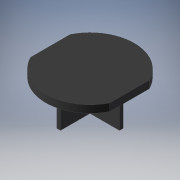
# Autodesk Inventor part: Syringe cap_Flat_Sides
Saved by Autodesk Inventor 2019 (Build 230136000, 136)
## iProperties
Created: 2019-01-24
Part Number: Syringe cap_Flat_Sides
Material: Generic
Document SubType Name: Modeling
Designer: dewanlab
Density: 1 g/cm^3
Appearance: Default
Author: dewanlab
Autodesk Inventor part; units mm, degrees
ref_plane "YZ Plane" through (0, 0, 0) normal (1, 0, 0) x (0, 1, 0)
ref_plane "XZ Plane" through (0, 0, 0) normal (0, 1, 0) x (-1, 0, 0)
ref_plane "XY Plane" through (0, 0, 0) normal (0, 0, 1) x (1, 0, 0)
sketch "Sketch1" plane through (0, 0, 0) normal (0, 1, 0) x (-1, 0, 0)
  line L0 (-17.05, 0) -> (-17.05, 8.4971)
  line L1 (-17.05, 0) -> (-17.05, -8.4971)
  line L2 (17.05, 0) -> (17.05, 8.4971)
  line L3 (17.05, 0) -> (17.05, -8.4971)
  arc A0 (-17.05, -8.4971) -> (17.05, -8.4971) centre (0, 0) ccw
  arc A1 (17.05, 8.4971) -> (-17.05, 8.4971) centre (0, 0) ccw
  constraints: 8 end point, 4 point on circle, 2 centre point, 2 point on line, 1 coincident
extrude "Extrusion1" add sketch "Sketch1" along normal blind 3.175
sketch "Sketch4" plane through (0, 0, 0) normal (0, -1, 0) x (-1, 0, 0)
  line L0 (-13.4937, -0.7938) -> (13.4938, -0.7938)
  line L1 (13.4938, -0.7938) -> (13.4938, 0.7938)
  line L2 (13.4938, 0.7938) -> (-13.4938, 0.7937)
  line L3 (-13.4938, 0.7937) -> (-13.4937, -0.7938)
  circle A0 centre (0, 0) radius 19.05 projected
  dimension "d16" = 26.9875
  dimension "d17" = 1.5875
  dimension "d18" = 18.2563
  dimension "d19" = 5.5563
  constraints: 8 end point, 2 parallel, 1 horizontal, 1 perpendicular
  measures "d16" distance of L1.end L2.end
  measures "d17" distance of L2.end L0.start
  measures "d18" distance edge to line of A0 L2
  measures "d19" distance edge to line of A0 L3
extrude "Extrusion3" add sketch "Sketch4" along normal blind 12.7 contours L3 L2 L1 L0
sketch "Sketch5" plane through (0, 0, 0) normal (0, -1, 0) x (-1, 0, 0)
  line L0 (13.4937, 0.7938) -> (-13.4938, 0.7937) projected
  line L1 (-0.7938, 0.7937) -> (0.6758, 0.7937)
  line L2 (0.6758, 0.7937) -> (0.6758, 13.4938)
  line L3 (0.6758, 13.4938) -> (-0.7938, 13.4938)
  line L4 (-0.7938, 13.4938) -> (-0.7938, 0.7937)
  line L5 (-13.4938, 0.7937) -> (-13.4937, -0.7938) projected
  point P0 (0, 0)
  dimension "d22" = 12.7
  dimension "d23" = 12.7
  constraints: 8 end point, 2 parallel, 1 horizontal, 1 perpendicular, 1 point on line
  measures "d22" distance of L3.end L1.start
  measures "d23" distance between parallel lines of L4 L5
extrude "Extrusion4" add sketch "Sketch5" along normal blind 12.7
sketch "Sketch7" plane through (0, 0, 0) normal (0, -1, 0) x (-1, 0, 0)
  line L0 (-13.4937, -0.7938) -> (13.4937, -0.7938) projected
  line L1 (-0.7938, -0.7938) -> (0.7937, -0.7938)
  line L2 (0.7937, -0.7938) -> (0.7937, -13.4938)
  line L3 (0.7937, -13.4938) -> (-0.7938, -13.4938)
  line L4 (-0.7938, -13.4938) -> (-0.7938, -0.7938)
  line L5 (13.4937, -0.7938) -> (13.4937, 0.7938) projected
  point P0 (0, 0)
  dimension "d28" = 12.7
  dimension "d29" = 1.5875
  dimension "d30" = 12.7
  constraints: 8 end point, 2 parallel, 1 horizontal, 1 perpendicular, 1 point on line
  measures "d28" distance of L1.end L2.end
  measures "d29" distance of L2.end L3.end
  measures "d30" distance between parallel lines of L5 L2
extrude "Extrusion5" add sketch "Sketch7" along normal blind 12.7
body "Solid1"
